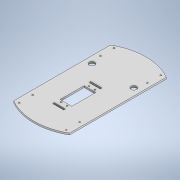
# Autodesk Inventor part: topPlate1
Saved by Autodesk Inventor 2020 (Build 240168000, 168)
## iProperties
Created: 2020-02-05
Part Number: topPlate1
Material: Generic
Document SubType Name: Modeling
Designer: mdjb501
Density: 1 g/cm^3
Appearance: Default
Author: mdjb501
Autodesk Inventor part; units mm, degrees
ref_plane "YZ Plane" through (0, 0, 0) normal (1, 0, 0) x (0, 1, 0)
ref_plane "XZ Plane" through (0, 0, 0) normal (0, 1, 0) x (-1, 0, 0)
ref_plane "XY Plane" through (0, 0, 0) normal (0, 0, 1) x (1, 0, 0)
sketch "Sketch1" plane through (0, 0, 0) normal (0, 1, 0) x (-1, 0, 0)
  line L0 (-50, 86.6025) -> (-50, -86.6025)
  line L1 (50, -86.6025) -> (50, 86.6025)
  arc A0 (50, 86.6025) -> (-50, 86.6025) centre (0, 0) ccw
  arc A1 (-50, -86.6025) -> (50, -86.6025) centre (0, 0) ccw
  circle A2 centre (42, -84.8528) radius 1.3
  circle A3 centre (42, -60.6528) radius 1.3
  circle A4 centre (-42, -84.8528) radius 1.3
  circle A5 centre (-42, -60.6528) radius 1.3
  circle A6 centre (42, 84.8528) radius 1.3
  circle A7 centre (42, 60.6528) radius 1.3
  circle A8 centre (-42, 84.8528) radius 1.3
  circle A9 centre (-42, 60.6528) radius 1.3
  circle A10 centre (37.5, -41.0117) radius 5
  circle A11 centre (-37.5, -41.0117) radius 5
  line L2 (10.5, 0) -> (10.5, 43)
  line L3 (10.5, 43) -> (-10.5, 43)
  line L4 (-10.5, 43) -> (-10.5, 0)
  line L5 (10.5, 0) -> (-10.5, 0)
  circle A12 centre (-5.4, -3.5) radius 1.3
  circle A13 centre (5.4, -3.5) radius 1.3
  circle A14 centre (5.4, 46.5) radius 1.3
  circle A15 centre (-5.4, 46.5) radius 1.3
  circle A16 centre (-2.7764, -36.0117) radius 16.406
  constraints: 17 centre point, 12 end point, 4 point on circle, 2 perpendicular, 1 coincident, 1 horizontal, 1 parallel, 1 vertical
extrude "Extrusion1" add sketch "Sketch1" against normal blind 3 contours A0 L1 A1 L0 | A16
sketch "Sketch2" plane through (0, 0, 0) normal (0, 1, 0) x (1, 0, 0)
  line L0 (-10.966, 9.168) -> (9.0417, 9.168)
  line L1 (9.0417, 9.168) -> (9.0417, 12.4204)
  line L2 (9.0417, 12.4204) -> (-10.966, 12.4204)
  line L3 (-10.966, 12.4204) -> (-10.966, 9.168)
  line L4 (-10.966, -53.1278) -> (9.0417, -53.1278)
  line L5 (9.0417, -53.1278) -> (9.0417, -56.1278)
  line L6 (9.0417, -56.1278) -> (-10.966, -56.1278)
  line L7 (-10.966, -56.1278) -> (-10.966, -53.1278)
  point P0 (0, 0)
  constraints: 16 end point, 6 perpendicular, 4 point on line, 1 horizontal
extrude "Extrusion2" cut sketch "Sketch2" against normal blind 3
body "Solid1"
